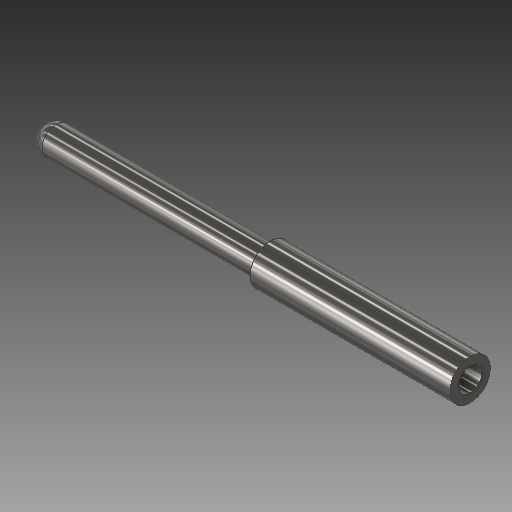
# Autodesk Inventor part: kls_pin
Saved by Autodesk Inventor 2019 (Build 230136000, 136)
## iProperties
Created: 2019-07-16
Part Number: kls_pin
Material: Сталь, нержавеющая, полированная
Document SubType Name: Modeling
Designer: Boss
Mass: 0.221243 g
Surface Area: 0.924466 cm^2
Volume: 0.0276553 cm^3
Density: 8 g/cm^3
Appearance: Нержавеющая — полированная
pin_small_rad: 0,600 мм
pin_big_dia: 1,700 мм
Author: Boss
Autodesk Inventor part; units mm, degrees
ref_plane "YZ Plane" through (0, 0, 0) normal (1, 0, 0) x (0, 1, 0)
ref_plane "XZ Plane" through (0, 0, 0) normal (0, 1, 0) x (-1, 0, 0)
ref_plane "XY Plane" through (0, 0, 0) normal (0, 0, 1) x (1, 0, 0)
sketch "Эскиз1" plane through (0, 0, 0) normal (0, 1, 0) x (-1, 0, 0)
  line L0 (16.8789, 0) -> (-16.2789, 0)
  arc A0 (16.2789, -0.6) -> (16.8789, 0) centre (16.2789, 0) ccw
  line L1 (16.2789, -0.6) -> (7.2789, -0.6)
  line L2 (7.2789, -0.6) -> (7.2789, -0.85)
  line L3 (7.2789, -0.85) -> (-1.1211, -0.85)
  line L4 (-1.1211, -0.85) -> (-1.1211, 0)
  point P0 (0, 0)
  point P1 (0, 0)
  dimension "pin_small_rad" = 0.6
  dimension "d1" = 18
  dimension "d2" = 9
  dimension "pin_big_dia" = 1.7
  constraints: 10 end point, 4 perpendicular, 3 point on line, 2 point on circle, 1 centre point, 1 coincident, 1 horizontal, 1 tangent
  measures "pin_small_rad" radius of A0
  measures "d1" distance from line of L0.start L4
  measures "d2" distance of L1.start L1.end
  measures "pin_big_dia" diameter of L3 L0
revolve "Вращение1" add sketch "Эскиз1" angle 360 about axis through (-16.8789, 0, 0) along (1, 0, 0)
hole "Отверстие1" at (1.1211, 0, 0) direction (-1, 0, 0) diameter 1 depth 2.5 tip angle 118
